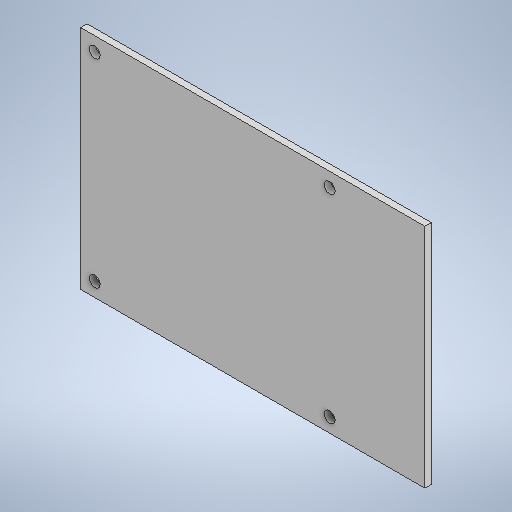
# Autodesk Inventor part: 라즈베리파이
Saved by Autodesk Inventor 2025 (Build 290162000, 162)
## iProperties
Created: 2024-06-01
Part Number: 라즈베리파이
Material: 일반
Document SubType Name: Modeling
Designer: ckhye
Density: 1 g/cm^3
Appearance: 기본값
Author: ckhye
Autodesk Inventor part; units mm, degrees
ref_plane "YZ Plane" through (0, 0, 0) normal (1, 0, 0) x (0, 1, 0)
ref_plane "XZ Plane" through (0, 0, 0) normal (0, 1, 0) x (-1, 0, 0)
ref_plane "XY Plane" through (0, 0, 0) normal (0, 0, 1) x (1, 0, 0)
sketch "스케치1" plane through (0, 0, 0) normal (0, 0, 1) x (1, 0, 0)
  line L0 (42.5, 28) -> (-42.5, 28)
  line L1 (-42.5, 28) -> (-42.5, -28)
  line L2 (-42.5, -28) -> (42.5, -28)
  line L3 (42.5, -28) -> (42.5, 28)
  line L4 (42.5, 28) -> (-42.5, -28) construction
  line L5 (-42.5, 28) -> (42.5, -28) construction
  line L6 (-72.7833, -24.5) -> (84.8355, -24.5) construction
  line L7 (-54.7439, 24.5) -> (74.9249, 24.5) construction
  line L8 (-39, 38.1575) -> (-39, -32.6978) construction
  line L9 (19, 25.9558) -> (19, -29.4685) construction
  circle A0 centre (-39, 24.5) radius 1.35
  circle A1 centre (19, 24.5) radius 1.35
  circle A2 centre (-39, -24.5) radius 1.35
  circle A3 centre (19, -24.5) radius 1.35
  point P0 (0, 0)
  dimension "d0" = 85
  dimension "d1" = 56
  dimension "d2" = 3.5
  dimension "d3" = 3.5
  dimension "d4" = 3.5
  dimension "d5" = 23.5
  dimension "d6" = 2.7
  dimension "d7" = 2.7
  dimension "d8" = 2.7
  dimension "d9" = 2.7
  constraints: 20 end point, 8 point on line, 4 centre point, 3 horizontal, 2 midpoint, 2 parallel, 2 vertical, 1 perpendicular
  measures "d0" distance of L2.end L1.end
  measures "d1" distance between parallel lines of L2 L0
  measures "d2" distance between parallel lines of L2 L6
  measures "d3" distance between parallel lines of L0 L7
  measures "d4" distance between parallel lines of L1 L8
  measures "d5" distance between parallel lines of L3 L9
  measures "d6" diameter of A0
  measures "d7" diameter of A1
  measures "d8" diameter of A2
  measures "d9" diameter of A3
extrude "돌출1" add sketch "스케치1" along normal blind 1.6
